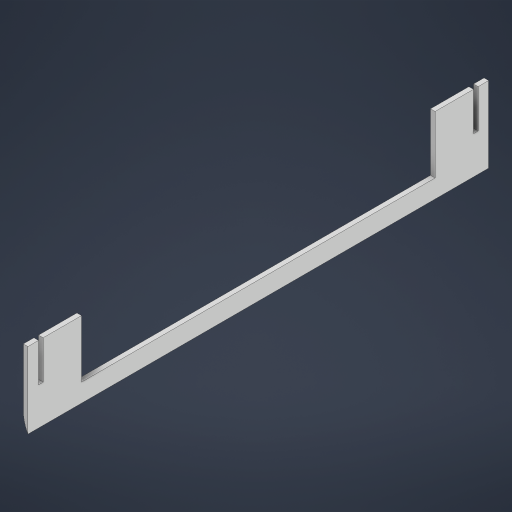
# Autodesk Inventor part: Battery_container_side
Saved by Autodesk Inventor 2024 (Build 280153000, 153)
## iProperties
Created: 2024-02-27
Part Number: Battery_container_side
Material: Generic
Document SubType Name: Modeling
Designer: calvi
Density: 1 g/cm^3
Appearance: Default
Author: calvi
Autodesk Inventor part; units mm, degrees
ref_plane "YZ Plane" through (0, 0, 0) normal (1, 0, 0) x (0, 1, 0)
ref_plane "XZ Plane" through (0, 0, 0) normal (0, 1, 0) x (-1, 0, 0)
ref_plane "XY Plane" through (0, 0, 0) normal (0, 0, 1) x (1, 0, 0)
sketch "Sketch1" plane through (0, 0, 0) normal (0, 0, 1) x (1, 0, 0)
  line L0 (25.4, 0) -> (146.304, 0)
  line L1 (171.704, 25.4) -> (171.704, 63.5)
  line L2 (171.704, 63.5) -> (0, 63.5)
  line L3 (0, 63.5) -> (0, 25.4)
  arc A0 (0, 25.4) -> (25.4, 0) centre (25.4, 25.4) ccw
  arc A1 (146.304, 0) -> (171.704, 25.4) centre (146.304, 25.4) ccw
  point P0 (0, 0)
  dimension "d0" = 171.704
  dimension "d2" = 50.8
  dimension "d3" = 50.8
  dimension "d4" = 63.5
  dimension "d5" = 63.5
  dimension "d6" = 0
  constraints: 8 end point, 4 point on circle, 4 tangent, 2 centre point, 2 parallel, 1 horizontal, 1 perpendicular
  measures "d0" distance of L2.end L1.end
  measures "d2" diameter of A0
  measures "d3" diameter of A1
  measures "d4" distance between parallel lines of L0 L2
  measures "d5" distance from line of L2 point (0, 0)
  measures "d6" distance from line of point (0, 0) L3
extrude "Extrusion1" add sketch "Sketch1" along normal blind 304.8
sketch "Sketch2" plane through (0, 0, 304.8) normal (0, 0, 1) x (1, 0, 0)
  line L0 (25.4, 0) -> (146.304, 0) projected
  line L1 (3.048, 63.5) -> (206.248, 63.5)
  line L2 (206.248, 63.5) -> (206.248, 0)
  line L3 (206.248, 0) -> (3.048, 0)
  line L4 (3.048, 0) -> (3.048, 63.5)
  line L5 (171.704, 63.5) -> (0, 63.5) projected
  line L6 (0, 63.5) -> (0, 25.4) projected
  point P0 (0, 0)
  dimension "d9" = 0
  dimension "d10" = 203.2
  dimension "d11" = 3.048
  constraints: 8 end point, 2 parallel, 1 horizontal, 1 perpendicular, 1 point on line
  measures "d9" distance between parallel lines of L5 L1
  measures "d10" distance between parallel lines of L2 L4
  measures "d11" distance between parallel lines of L6 L4
extrude "Extrusion2" cut sketch "Sketch2" against normal through all
sketch "Sketch5" plane through (0, 25.4, 0) normal (-1, 0, 0) x (0, 0, 1)
  line L0 (6.985, 38.1) -> (10.033, 38.1)
  line L1 (10.033, 38.1) -> (10.033, 12.7)
  line L2 (10.033, 12.7) -> (6.985, 12.7)
  line L3 (6.985, 12.7) -> (6.985, 38.1)
  line L4 (0, 38.1) -> (304.8, 38.1) projected
  line L5 (0, 38.1) -> (0, 0) projected
  line L6 (152.4, 38.1) -> (152.4, 0)
  line L7 (0, 0) -> (304.8, 0) projected
  line L8 (297.815, 38.1) -> (294.767, 38.1)
  line L9 (294.767, 38.1) -> (294.767, 12.7)
  line L10 (294.767, 12.7) -> (297.815, 12.7)
  line L11 (297.815, 12.7) -> (297.815, 38.1)
  line L12 (304.8, 38.1) -> (0, 38.1)
  line L13 (304.8, 38.1) -> (304.8, 0)
  point P0 (0, -25.4)
  point P1 (297.815, 38.1)
  point P2 (294.767, 38.1)
  dimension "d22" = 3.048
  dimension "d23" = 25.4
  dimension "d24" = 0
  dimension "d25" = 6.985
  constraints: 22 end point, 6 symmetric about line, 2 midpoint, 2 parallel, 1 horizontal, 1 perpendicular
  measures "d22" distance of L1.end L2.end
  measures "d23" distance of L0.end L1.end
  measures "d24" distance between parallel lines of L4 L0
  measures "d25" distance between parallel lines of L5 L3
extrude "Extrusion5" cut sketch "Sketch5" against normal through all contours L0 L1 L2 L3 | L4 L11 L10 L9
sketch "Sketch6" plane through (0, 25.4, 0) normal (-1, 0, 0) x (0, 0, 1)
  line L0 (10.033, 38.1) -> (294.767, 38.1) projected
  line L1 (0, 0) -> (304.8, 0) projected
  line L2 (35.433, 38.1) -> (269.367, 38.1)
  line L3 (269.367, 38.1) -> (269.367, 0)
  line L4 (269.367, 0) -> (35.433, 0)
  line L5 (35.433, 0) -> (35.433, 38.1)
  line L6 (10.033, 38.1) -> (10.033, 12.7) projected
  line L7 (294.767, 12.7) -> (294.767, 38.1) projected
  point P0 (0, -25.4)
  point P1 (35.433, 0)
  dimension "d28" = 25.4
  dimension "d29" = 25.4
  constraints: 8 end point, 2 parallel, 2 point on line, 1 horizontal, 1 perpendicular
  measures "d28" distance between parallel lines of L5 L6
  measures "d29" distance between parallel lines of L7 L3
extrude "Extrusion6" cut sketch "Sketch6" against normal through all
body "Solid1"
